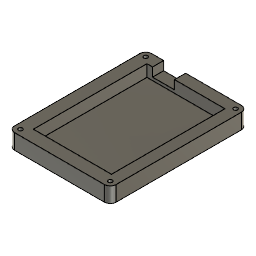
Case_Bottom (Autodesk Fusion 360 design; units mm, degrees)
part number: 2025-12-31-23-33-16-978
Autodesk Fusion 360 part; units mm, degrees
sketch "Sketch1" plane through (0, 0, 0) normal (0, 0, 1) x (1, 0, 0)
  line L0 (0, 0) -> (66, 0)
  line L1 (66, 0) -> (66, 96)
  line L2 (66, 96) -> (0, 96)
  line L3 (0, 96) -> (0, 0)
  line L4 (-10.5, -10.5) -> (75.5, -10.5)
  line L5 (75.5, -10.5) -> (75.5, 105.5)
  line L6 (75.5, 105.5) -> (-10.5, 105.5)
  line L7 (-10.5, 105.5) -> (-10.5, -10.5)
  circle A0 centre (-5.5, 100.5) radius 1.7
  circle A1 centre (70.5, 100.5) radius 1.7
  circle A2 centre (70.5, -5.5) radius 1.7
  circle A3 centre (-5.5, -5.5) radius 1.7
  circle A4 centre (-5.5, 100.5) radius 3
  circle A5 centre (70.5, 100.5) radius 3
  circle A6 centre (-5.5, -5.5) radius 3
  circle A7 centre (70.5, -5.5) radius 3
  dimension "d1" = 66
  dimension "d2" = 96
  dimension "d3" = 86
  dimension "d4" = 116
  dimension "d5" = 9.5
  dimension "d6" = 9.5
  dimension "d7" = 3.4
  dimension "d8" = 5
  dimension "d9" = 5
  dimension "d10" = 3.4
  dimension "d11" = 5
  dimension "d12" = 5
  dimension "d13" = 3.4
  dimension "d14" = 5
  dimension "d15" = 5
  dimension "d16" = 3.4
  dimension "d17" = 5
  dimension "d18" = 5
  dimension "d19" = 6
  dimension "d20" = 5
  dimension "d21" = 5
  dimension "d22" = 6
  dimension "d23" = 5
  dimension "d24" = 5
  dimension "d25" = 6
  dimension "d26" = 5
  dimension "d27" = 5
  dimension "d28" = 6
  dimension "d29" = 5
  dimension "d30" = 5
  constraint horizontal L0
  constraint vertical L1
  constraint horizontal L2
  constraint vertical L3
  constraint coincident L0.start L3.end
  constraint horizontal L4
  constraint vertical L5
  constraint horizontal L6
  constraint vertical L7
  measures "d1" distance of L0.start L0.end
  measures "d2" distance of L0.start L2.end
  measures "d3" distance of L4.start L4.end
  measures "d4" distance of L4.start L6.end
  measures "d5" distance of L2 L6
  measures "d6" distance of L1 L5
  measures "d7" diameter of A0
  measures "d8" distance of L6 A0.centre
  measures "d9" distance of L7 A0.centre
  measures "d10" diameter of A1
  measures "d11" distance of L6 A1.centre
  measures "d12" distance of L5 A1.centre
  measures "d13" diameter of A2
  measures "d14" distance of L5 A2.centre
  measures "d15" distance of L4 A2.centre
  measures "d16" diameter of A3
  measures "d17" distance of L4 A3.centre
  measures "d18" distance of L7 A3.centre
  measures "d19" diameter of A4
  measures "d20" distance of L6 A0.centre
  measures "d21" distance of L7 A0.centre
  measures "d22" diameter of A5
  measures "d23" distance of L6 A1.centre
  measures "d24" distance of L5 A1.centre
  measures "d25" diameter of A6
  measures "d26" distance of L4 A3.centre
  measures "d27" distance of L7 A3.centre
  measures "d28" diameter of A7
  measures "d29" distance of L5 A2.centre
  measures "d30" distance of L4 A2.centre
extrude "Extrude1" add sketch "Sketch1" along normal blind 9.9 from surface at 3.1 contours A4 | A5 | A6 | A7 makes body 1 at (71.3125, 103.3879, 9.7) makes body 2 at (-2.5037, -5.6495, 9.7) makes body 3 at (-2.6809, 99.4739, 9.7) makes body 4 at (73.4963, -5.6495, 9.7)
extrude "Extrude2" add sketch "Sketch1" along normal blind 13 contours L4 L5 L6 L7 bodies 1 2 3 4
extrude "Extrude3" add sketch "Sketch1" along normal blind 3 contours L0 L1 L2 L3 bodies 1
sketch "Sketch2" plane through (0, 0, 13) normal (0, 0, 1) x (-1, 0, 0)
  circle A0 centre (-70.5, -100.5) radius 1.7
  circle A1 centre (-70.5, 5.5) radius 1.7
  line L0 (0, 0) -> (0, -96)
  line L1 (0, -96) -> (-66, -96)
  line L2 (-66, -96) -> (-66, 0)
  line L3 (-66, 0) -> (0, 0)
  line L4 (10.5, -105.5) -> (10.5, 10.5)
  line L5 (10.5, 10.5) -> (-75.5, 10.5)
  line L6 (-75.5, 10.5) -> (-75.5, -105.5)
  line L7 (-75.5, -105.5) -> (10.5, -105.5)
  circle A2 centre (5.5, 5.5) radius 1.7
  circle A3 centre (5.5, -100.5) radius 1.7
sketch "Sketch3" plane through (0, 0, 13) normal (0, 0, 1) x (1, 0, 0)
  line L0 (4.75, 96) -> (23.25, 96)
  line L1 (23.25, 96) -> (23.25, 105.5)
  line L2 (23.25, 105.5) -> (4.75, 105.5)
  line L3 (4.75, 105.5) -> (4.75, 96)
  line L4 (-10.5, 105.5) -> (-10.5, -10.5)
  dimension "d38" = 18.5
  dimension "d39" = 9.5
  dimension "d40" = 15.25
  constraint horizontal L0
  constraint vertical L1
  constraint horizontal L2
  constraint vertical L3
  measures "d38" distance of L0.start L0.end
  measures "d39" distance of L0.start L2.end
  measures "d40" distance of L3 L4
extrude "Extrude4" cut sketch "Sketch3" against normal blind 7.5 bodies 1
fillet "Fillet1" radius 5 1 edges at (75.5, -10.5, 6.5) on bodies 1
fillet "Fillet2" radius 5 3 edges at (75.5, 105.5, 6.5) (-10.5, 105.5, 6.5) (-10.5, -10.5, 6.5) on bodies 1
sketch "Sketch4" plane through (0, 0, 0) normal (0, 0, 1) x (1, 0, 0)
  line L0 (68, 92) -> (3, 92) construction
  line L1 (3, 92) -> (3, 97) construction
  line L2 (3, 97) -> (68, 97) construction
  line L3 (68, 97) -> (68, 92) construction
  dimension "d47" = 5
  text T0 "Saim ModuPad" font "Arial" height 5 bold align centre middle in box 65 x 5 at (68, 92) x (-1, 0) y (0, 1) spacing 1
extrude "Extrude5" add sketch "Sketch4" against normal blind 0.2 text T0 bodies 1
equation "d48 = 'Saim ModuPad'"
